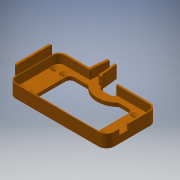
# Autodesk Inventor part: Phone_Cas
Saved by Autodesk Inventor 2017 (Build 210142000, 142)
## iProperties
Created: 2015-11-17
Part Number: Phone_Cas
Material: Generic
Document SubType Name: Modeling
Designer: Team Titanium
Density: 1 g/cm^3
Appearance: Orange
Author: Team Titanium
Autodesk Inventor part; units mm, degrees
ref_plane "YZ Plane" through (0, 0, 0) normal (1, 0, 0) x (0, 1, 0)
ref_plane "XZ Plane" through (0, 0, 0) normal (0, 1, 0) x (-1, 0, 0)
ref_plane "XY Plane" through (0, 0, 0) normal (0, 0, 1) x (1, 0, 0)
sketch "Sketch1" plane through (0, 0, 0) normal (0, 1, 0) x (-1, 0, 0)
  line L0 (67.1674, 24.5628) -> (-66.5636, 24.5628)
  line L1 (-66.5636, 24.5628) -> (-66.5636, -42.8742)
  line L2 (-66.5636, -42.8742) -> (67.1674, -42.8742)
  line L3 (67.1674, -42.8742) -> (67.1674, 24.5628)
  line L4 (69.1994, 26.5948) -> (-68.5956, 26.5948)
  line L5 (-68.5956, 26.5948) -> (-68.5956, -44.9062)
  line L6 (-68.5956, -44.9062) -> (69.1994, -44.9062)
  line L7 (69.1994, -44.9062) -> (69.1994, 26.5948)
  point P0 (0, 0)
  dimension "d0" = 133.731
  dimension "d1" = 67.437
  dimension "d2" = 2.032
  constraints: 16 end point, 4 parallel, 2 perpendicular, 1 horizontal, 3 other
  measures "d0" distance of L1.end L2.end
  measures "d1" distance of L2.end L0.start
  measures "d2" distance between parallel lines of L4 L0
extrude "Extrusion1" add sketch "Sketch1" along normal blind 12.7
sketch "Sketch2" plane through (0, 0, 0) normal (0, -1, 0) x (1, 0, 0)
  line L0 (68.5956, 26.5948) -> (68.5956, -44.9062) projected
  line L1 (68.5956, -44.9062) -> (-69.1994, -44.9062) projected
  line L2 (-69.1994, -44.9062) -> (-69.1994, 26.5948) projected
  line L3 (-69.1994, 26.5948) -> (68.5956, 26.5948) projected
  point P0 (0, 0)
extrude "Extrusion2" add sketch "Sketch2" along normal blind 5.08
fillet "Fillet1" radius 7.62 4 edges at (-67.1674, 6.35, -42.8742) (66.5636, 6.35, -42.8742) (-67.1674, 6.35, 24.5628) (66.5636, 6.35, 24.5628)
fillet "Fillet2" radius 10.795 4 edges at (-69.1994, 3.81, -44.9062) (68.5956, 3.81, -44.9062) (68.5956, 3.81, 26.5948) (-69.1994, 3.81, 26.5948)
sketch "Sketch3" plane through (0, 12.7, 0) normal (0, 1, 0) x (1, 0, 0)
  line L0 (57.8006, 44.9062) -> (-58.4044, 44.9062) projected
  line L1 (-59.5474, 42.8742) -> (58.9436, 42.8742) projected
  line L2 (-23.4286, 44.9062) -> (-12.7606, 44.9062)
  line L3 (-12.7606, 44.9062) -> (-12.7606, 42.8742)
  line L4 (-12.7606, 42.8742) -> (-23.4286, 42.8742)
  line L5 (-23.4286, 42.8742) -> (-23.4286, 44.9062)
  line L6 (-67.1674, -16.9428) -> (-67.1674, 35.2542) projected
  point P0 (0, 0)
  point P1 (-18.0946, 42.8742)
  dimension "d9" = 10.668
  dimension "d50" = 49.0728
  constraints: 8 end point, 2 parallel, 2 point on line, 1 horizontal, 1 midpoint, 1 perpendicular
  measures "d9" distance of L2.start L2.end
  measures "d50" distance from line of point (-18.095, 42.874) L6
extrude "Extrusion3" cut sketch "Sketch3" against normal up to surface (12.7 mm away)
sketch "Sketch4" plane through (0, 12.7, 0) normal (0, 1, 0) x (1, 0, 0)
  line L0 (-12.7606, 44.9062) -> (-12.7606, 50.6847)
  line L1 (-12.7606, 50.6847) -> (-14.8579, 67.7662)
  line L2 (-23.4286, 44.9062) -> (-23.4286, 50.6847)
  line L3 (-23.4286, 50.6847) -> (-21.3312, 67.7662)
  line L4 (-23.4286, 44.9062) -> (-58.4044, 44.9062) projected
  line L5 (-14.8579, 67.7662) -> (-11.6591, 67.7662)
  line L6 (-11.6591, 67.7662) -> (-9.5856, 50.8788)
  line L7 (57.8006, 44.9062) -> (-12.7606, 44.9062) projected
  line L8 (-9.5856, 44.9062) -> (-9.5856, 50.8788)
  line L9 (-21.3312, 67.7662) -> (-24.5301, 67.7662)
  line L10 (-24.5301, 67.7662) -> (-26.6036, 50.8788)
  line L11 (-26.6036, 50.8788) -> (-26.6036, 44.9062)
  line L12 (-67.1674, -16.9428) -> (-67.1674, 35.2542) projected
  point P0 (0, 0)
  dimension "d14" = 5.7785
  dimension "d15" = 22.86
  dimension "d17" = 3.175
  dimension "d18" = 3.175
  dimension "d19" = 3.175
  dimension "d20" = 3.175
  dimension "d45" = 173
  dimension "d46" = 173
  dimension "d47" = 6.4733
  constraints: 20 end point, 2 horizontal, 2 horizontal alignment, 2 perpendicular, 2 point on line, 2 vertical, 1 equal length, 1 parallel
  measures "d14" distance of L2.start L2.end
  measures "d15" distance from line of L3.end L4
  measures "d17" distance between parallel lines of L6 L1
  measures "d18" distance between parallel lines of L8 L0
  measures "d19" distance between parallel lines of L3 L10
  measures "d20" distance between parallel lines of L2 L11
  measures "d45" angle of L2 L3
  measures "d46" angle of L0 L1
  measures "d47" distance of L1.end L3.end
extrude "Extrusion4" add sketch "Sketch4" against normal up to surface (12.7 mm away)
sketch "Sketch5" plane through (0, -5.08, 0) normal (0, -1, 0) x (1, 0, 0)
  line L0 (-58.4044, -44.9062) -> (57.8006, -44.9062) projected
  line L1 (-26.6036, -50.8788) -> (-26.6036, -44.9062) projected
  line L2 (-24.5301, -67.7662) -> (-26.6036, -50.8788) projected
  line L3 (-9.5856, -50.8788) -> (-11.6591, -67.7662) projected
  line L4 (-9.5856, -44.9062) -> (-9.5856, -50.8788) projected
  line L5 (-24.5301, -67.7662) -> (-11.6591, -67.7662)
  point P0 (0, 0)
  constraints: 2 end point, 1 horizontal
extrude "Extrusion5" add sketch "Sketch5" against normal up to surface (5.08 mm away)
fillet "Fillet3" radius 1.524 2 edges at (-12.7606, 6.35, -42.8742) (-23.4286, 6.35, -42.8742)
fillet "Fillet4" radius 1.524 2 edges at (-26.6036, 3.81, -44.9062) (-9.5856, 3.81, -44.9062)
fillet "Fillet5" radius 1.016 15 edges at (-64.9355, 12.7, 22.331) (-67.1674, 12.7, -9.1557) (-64.9355, 12.7, -40.6423) (-42.25, 12.7, -42.8742) (-23.875, 12.7, -43.3205) (-23.4286, 12.7, -47.5414) (64.3318, 12.7, 22.331) (66.5636, 12.7, -9.1557) (64.3318, 12.7, -40.6423) (23.8535, 12.7, -42.8742) (-12.3142, 12.7, -43.3205) (-12.7606, 12.7, -47.5414) (-0.3019, 12.7, 24.5628) (-13.8093, 12.7, -59.2254) (-22.3799, 12.7, -59.2254)
sketch "Sketch6" plane through (0, 12.7, 0) normal (0, 1, 0) x (1, 0, 0)
  line L0 (-8.0616, 44.9062) -> (57.8006, 44.9062) projected
  line L1 (12.8426, 44.9062) -> (-7.4774, 44.9062)
  line L2 (-7.4774, 44.9062) -> (-7.4774, 38.5562)
  line L3 (-7.4774, 38.5562) -> (12.8426, 38.5562)
  line L4 (12.8426, 38.5562) -> (12.8426, 44.9062)
  line L5 (57.8006, -26.5948) -> (-58.4044, -26.5948) projected
  line L6 (-67.1674, -16.9428) -> (-67.1674, 35.2542) projected
  point P0 (0, 0)
  point P1 (2.6826, 38.5562)
  dimension "d29" = 6.35
  dimension "d30" = 69.85
  dimension "d61" = 20.32
  constraints: 8 end point, 2 parallel, 1 horizontal, 1 midpoint, 1 perpendicular, 1 point on line
  measures "d29" distance between parallel lines of L3 L0
  measures "d30" distance from line of point (2.683, 38.556) L6
  measures "d61" distance of L2.end L3.end
extrude "Extrusion6" cut sketch "Sketch6" against normal through all
fillet "Fillet6" radius 4.064 2 edges at (12.8426, -2.54, -38.5562) (-7.4774, -2.54, -38.5562)
sketch "Sketch7" plane through (0, 0, 0) normal (0, 1, 0) x (1, 0, 0)
  line L0 (60.4676, 41.2012) -> (60.4676, -21.2651)
  line L1 (50.9426, -21.2651) -> (50.9426, 41.2012)
  line L2 (-60.8174, 33.3314) -> (-60.8174, -18.2808)
  line L3 (-51.2924, 33.532) -> (-51.2924, -18.0802)
  line L4 (-67.1674, -17.4508) -> (-67.1674, 35.2542) projected
  circle A0 centre (62.0551, 32.0157) radius 1.5875
  circle A1 centre (62.0551, -13.7043) radius 1.5875
  circle A2 centre (49.3551, -13.7043) radius 1.5875
  circle A3 centre (49.3551, 32.0157) radius 1.5875
  line L5 (66.5636, -16.9428) -> (66.5636, 35.2542) projected
  circle A4 centre (-49.7049, 32.0157) radius 1.5875
  circle A5 centre (-62.4049, 32.0157) radius 1.5875
  circle A6 centre (-49.7049, -13.7043) radius 1.5875
  circle A7 centre (-62.4049, -13.7043) radius 1.5875
  point P0 (0, 0)
  point P1 (66.5636, 9.1557)
  dimension "d34" = 9.525
  dimension "d35" = 9.525
  dimension "d36" = 111.76
  dimension "d37" = 6.35
  dimension "d38" = 22.86
  dimension "d39" = 22.86
  dimension "d40" = 3.175
  constraints: 8 centre point, 8 end point, 8 tangent, 7 equal radius, 6 horizontal alignment, 3 vertical, 1 midpoint
  measures "d34" distance between parallel lines of L0 L1
  measures "d35" distance between parallel lines of L3 L2
  measures "d36" distance between parallel lines of L2 L1
  measures "d37" distance between parallel lines of L2 L4
  measures "d38" vertical distance of A0.centre point (66.564, 9.156)
  measures "d39" vertical distance of A1.centre point (66.564, 9.156)
  measures "d40" diameter of A0
extrude "Extrusion7" cut sketch "Sketch7" against normal through all
sketch "Sketch8" plane through (0, 0, 0) normal (0, 1, 0) x (1, 0, 0)
  line L0 (-44.3074, -16.9428) -> (43.7036, -16.9428)
  line L1 (43.7036, -16.9428) -> (43.7036, 35.2542)
  line L2 (43.7036, 35.2542) -> (-44.3074, 35.2542)
  line L3 (-44.3074, 35.2542) -> (-44.3074, -16.9428)
  line L4 (-67.1674, -16.9428) -> (-67.1674, 35.2542) projected
  line L5 (66.5636, 35.2542) -> (66.5636, -16.9428) projected
  line L6 (58.9436, -24.5628) -> (-59.5474, -24.5628) projected
  line L7 (-11.2366, 42.8742) -> (58.9436, 42.8742) projected
  point P0 (0, 0)
  point P1 (12.8426, -24.5628)
  point P2 (12.8426, 42.8742)
  dimension "d53" = 22.86
  dimension "d54" = 22.86
  dimension "d55" = 7.62
  dimension "d56" = 7.62
  constraints: 8 end point, 2 parallel, 1 horizontal, 1 perpendicular
  measures "d53" distance between parallel lines of L3 L4
  measures "d54" distance between parallel lines of L1 L5
  measures "d55" distance between parallel lines of L0 L6
  measures "d56" distance between parallel lines of L2 L7
extrude "Extrusion8" cut sketch "Sketch8" against normal through all
fillet "Fillet7" radius 6.35 4 edges at (-44.3074, -2.54, -35.2542) (-44.3074, -2.54, 16.9428) (43.7036, -2.54, 16.9428) (43.7036, -2.54, -35.2542)
sketch "Sketch10" plane through (0, 0, 0) normal (0, 1, 0) x (1, 0, 0)
  line L0 (-37.9574, -16.9428) -> (37.3536, -16.9428) projected
  line L1 (37.3536, 35.2542) -> (-37.9574, 35.2542) projected
  arc A0 (-18.5377, 35.2542) -> (23.6849, 35.2542) centre (2.5736, 56.3248) ccw
  point P0 (0, 0)
  constraints: 2 point on circle, 2 point on line, 1 centre point
extrude "Extrusion10" add sketch "Sketch10" against normal up to surface (5.08 mm away)
sketch "Sketch11" plane through (0, 12.7, 0) normal (0, 1, 0) x (1, 0, 0)
  line L0 (64.9731, -8.3068) -> (68.5956, -8.3068)
  line L1 (68.5956, -8.3068) -> (68.5956, 3.8852)
  line L2 (68.5956, 3.8852) -> (64.9731, 3.8852)
  line L3 (64.9731, 3.8852) -> (64.9731, -8.3068)
  line L4 (58.9436, -24.5628) -> (-59.5474, -24.5628) projected
  line L5 (68.5956, -15.7998) -> (68.5956, 34.1112) projected
  point P0 (0, 0)
  point P1 (64.9731, -2.2108)
  dimension "d62" = 12.192
  dimension "d63" = 22.352
  dimension "d72" = 0
  constraints: 8 end point, 2 parallel, 1 horizontal, 1 midpoint, 1 perpendicular
  measures "d62" distance of L2.end L0.start
  measures "d63" distance from line of L4 point (64.973, -2.211)
  measures "d72" distance between parallel lines of L5 L1
extrude "Extrusion11" cut sketch "Sketch11" against normal blind 7.62
chamfer "Chamfer1" distance 3.175 angle 45 8 edges at (47.7676, 0, -32.0157) (47.7676, 0, 13.7043) (-51.2924, 0, 13.7043) (-63.9924, 0, 13.7043) (-51.2924, 0, -32.0157) (-63.9924, 0, -32.0157) (60.4676, 0, -32.0157) (60.4676, 0, 13.7043)
sketch "Sketch13" plane through (0, 12.7, 0) normal (0, 1, 0) x (1, 0, 0)
  line L0 (20.9706, -25.5788) -> (46.3706, -25.5788)
  line L1 (46.3706, -25.5788) -> (46.3706, -24.5628)
  line L2 (46.3706, -24.5628) -> (20.9706, -24.5628)
  line L3 (20.9706, -24.5628) -> (20.9706, -25.5788)
  line L4 (-59.5474, -24.5628) -> (58.9436, -24.5628) projected
  line L5 (68.5956, -15.7998) -> (68.5956, -8.3068) projected
  line L6 (-58.4044, -26.5948) -> (57.8006, -26.5948) projected
  point P0 (0, 0)
  dimension "d73" = 0
  dimension "d74" = 22.225
  dimension "d75" = 25.4
  dimension "d77" = 1.016
  constraints: 8 end point, 2 parallel, 1 horizontal, 1 perpendicular
  measures "d73" distance between parallel lines of L4 L2
  measures "d74" distance between parallel lines of L5 L1
  measures "d75" distance between parallel lines of L3 L1
  measures "d77" distance between parallel lines of L6 L0
extrude "Extrusion13" cut sketch "Sketch13" against normal up to surface (12.7 mm away)
thicken "Thicken1" operation add thickness 12.7 both sides no extend neighbours yes toward (-1, 0, 0) faces at (20.9706, 8.128, 25.2402)
sketch "Sketch14" plane through (-69.1994, -5.08, 15.7998) normal (-1, 0, 0) x (0, 0, 1)
  line L0 (0, 17.78) -> (0, 0) projected
  line L1 (-49.911, 17.78) -> (0, 17.78) projected
  line L2 (-49.911, 0) -> (-49.911, 17.78) projected
  line L3 (0, 0) -> (-49.911, 0) projected
  point P0 (-15.7998, 5.08)
extrude "Extrusion14" add sketch "Sketch14" along normal blind 2.54
sketch "Sketch15" plane through (0, 12.7, 0) normal (0, 1, 0) x (1, 0, 0)
  line L0 (68.5956, -8.3068) -> (67.5796, -8.3068) projected
  line L1 (67.5796, -16.9428) -> (67.5796, -8.3068) projected
  arc A0 (58.9436, -25.5788) -> (67.5796, -16.9428) centre (58.9436, -16.9428) ccw projected
  line L2 (46.3706, -25.5788) -> (58.9436, -25.5788) projected
  line L3 (8.2706, -25.5788) -> (46.3706, -25.5788) projected
  line L4 (-59.5474, -25.5788) -> (8.2706, -25.5788) projected
  arc A1 (-68.1834, -16.9428) -> (-59.5474, -25.5788) centre (-59.5474, -16.9428) ccw projected
  line L5 (-68.1834, 35.2542) -> (-68.1834, -16.9428) projected
  arc A2 (-59.5474, 43.8902) -> (-68.1834, 35.2542) centre (-59.5474, 35.2542) ccw projected
  line L6 (-24.9526, 43.8902) -> (-59.5474, 43.8902) projected
  arc A3 (-24.9526, 43.8902) -> (-24.4446, 44.3982) centre (-24.9526, 44.3982) ccw projected
  line L7 (-24.4446, 50.7468) -> (-24.4446, 44.3982) projected
  line L8 (-22.3549, 67.7662) -> (-24.4446, 50.7468) projected
  line L9 (-22.3549, 67.7662) -> (-24.5301, 67.7662) projected
  line L10 (-24.5301, 67.7662) -> (-26.6036, 50.8788) projected
  line L11 (-26.6036, 50.8788) -> (-26.6036, 46.4302) projected
  arc A4 (-28.1276, 44.9062) -> (-26.6036, 46.4302) centre (-28.1276, 46.4302) ccw projected
  line L12 (-28.1276, 44.9062) -> (-58.4044, 44.9062) projected
  arc A5 (-58.4044, 44.9062) -> (-69.1994, 34.1112) centre (-58.4044, 34.1112) ccw projected
  line L13 (-69.1994, 34.1112) -> (-71.7394, 34.1112) projected
  line L14 (-71.7394, -15.7998) -> (-71.7394, 34.1112) projected
  line L15 (-69.1994, -15.7998) -> (-71.7394, -15.7998) projected
  arc A6 (-69.1994, -15.7998) -> (-58.4044, -26.5948) centre (-58.4044, -15.7998) ccw projected
  line L16 (-58.4044, -26.5948) -> (57.8006, -26.5948) projected
  arc A7 (57.8006, -26.5948) -> (68.5956, -15.7998) centre (57.8006, -15.7998) ccw projected
  line L17 (68.5956, -15.7998) -> (68.5956, -8.3068) projected
  line L18 (-71.7394, 34.1112) -> (-71.7394, -15.7998) projected
  line L19 (-68.1834, 35.2542) -> (-68.1834, -16.9428) projected
  line L20 (-71.7394, 34.1112) -> (-68.1834, 34.1112)
  line L21 (-68.1834, 34.1112) -> (-68.1834, -15.7998)
  line L22 (-68.1834, -15.7998) -> (-71.7394, -15.7998)
  line L23 (-71.7394, -15.7998) -> (-71.7394, 34.1112)
  point P0 (0, 0)
  constraints: 8 end point, 2 parallel, 1 horizontal, 1 perpendicular, 1 point on line
extrude "Extrusion15" add sketch "Sketch15" along normal blind 12.7 contours L15 L14 L13 L20 L5 L22
fillet "Fillet8" radius 2.54 2 edges at (-71.7394, 10.16, 15.7998) (-71.7394, 10.16, -34.1112)
fillet "Fillet9" radius 1.27 5 edges at (-70.9954, 25.4, 15.0559) (-71.7394, 25.4, -9.1557) (-70.9954, 25.4, -33.3672) (-68.6914, 25.4, -34.1112) (-68.6914, 25.4, 15.7998)
sketch "Sketch12" plane through (0, 0, 0) normal (0, 1, 0) x (1, 0, 0)
  line L0 (-37.1264, 29.2031) -> (-37.1264, 48.6718)
  line L1 (-37.1264, 48.6718) -> (-76.0638, 48.6718)
  line L2 (-76.0638, 48.6718) -> (-76.0638, -33.2779)
  line L3 (-76.0638, -33.2779) -> (73.5736, -33.2779)
  line L4 (73.5736, -33.2779) -> (73.5736, -28.0712)
  line L5 (73.5736, -28.0712) -> (56.8215, -28.0712)
  line L6 (56.8215, -28.0712) -> (56.8215, 13.3564)
  line L7 (56.8215, 13.3564) -> (73.5736, 13.3564)
  line L8 (73.5736, 13.3564) -> (73.5736, 51.8411)
  line L9 (73.5736, 51.8411) -> (0, 53.4258)
  line L10 (0, 53.4258) -> (0, 21.4966)
  line L11 (0, 21.4966) -> (-37.1264, 29.2031)
  point P0 (0, 0)
  constraints: 24 end point, 7 perpendicular, 2 point on line, 1 parallel, 1 vertical
body "Solid1"
